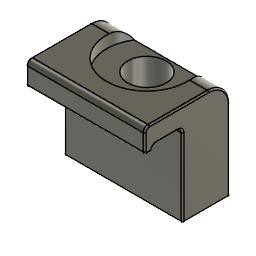
PhoneSupportTop (Autodesk Fusion 360 design; units mm, degrees)
part number: 2026-05-26-19-53-29-844
Autodesk Fusion 360 part; units mm, degrees
sketch "PhoneSupportTop" plane through (0, 0, 0) normal (1, 0, 0) x (0, 1, 0)
  line L0 (0, 0) -> (20, 0)
  line L1 (0, 33) -> (0, 0)
  line L2 (-2, 35) -> (-11, 35)
  line L3 (-13.4495, 33) -> (-15, 33)
  line L4 (-16, 34) -> (-16, 41)
  arc A0 (-11, 35) -> (-12.9596, 33.4) centre (-11, 33) ccw
  arc A1 (0, 33) -> (-2, 35) centre (-2, 33) ccw
  line L5 (-14, 43) -> (11, 43)
  line L6 (20, 0) -> (20, 34)
  arc A2 (20, 34) -> (11, 43) centre (11, 34) ccw
  arc A3 (-14, 43) -> (-16, 41) centre (-14, 41) ccw
  arc A4 (-13.4495, 33) -> (-12.9596, 33.4) centre (-13.4495, 33.5) ccw
  arc A5 (-16, 34) -> (-15, 33) centre (-15, 34) ccw
  point P0 (-13, 33)
  point P1 (-16, 33)
  point P2 (-16, 43)
  dimension "d3" = 20
  dimension "d7" = 4
  dimension "d8" = 3
  dimension "d10" = 2
  dimension "d11" = 9
  dimension "d13" = 34
  dimension "d14" = 27
  dimension "d15" = 10
  dimension "d16" = 9
  dimension "d17" = 2
  dimension "d18" = 0.5
  dimension "d19" = 1
  constraint horizontal L0
  constraint vertical L1
  constraint coincident L0.start L1.end
  constraint perpendicular L1 L2
  constraint horizontal L3
  constraint perpendicular L3 L4
  constraint tangent L1 A1
  constraint tangent L2 A1
  constraint perpendicular L5 L6
  constraint tangent L6 A2
  constraint tangent L5 A2
  constraint coincident P2 L4
  constraint coincident P2 L5
  constraint tangent L4 A3
  constraint tangent L5 A3
  constraint coincident P0 L3
  constraint coincident P0 A0
  constraint tangent L3 A4
  constraint tangent A0 A4
  constraint coincident P1 L3
  constraint coincident P1 L4
  constraint tangent L3 A5
  constraint tangent L4 A5
  measures "d3" distance of L0.start L0.end
  measures "d7" diameter of A0
  measures "d8" distance of P0 P1
  measures "d10" radius of A1
  measures "d11" radius of A2
  measures "d13" distance of L0.end L6.end
  measures "d14" distance of P2 L5.end
  measures "d15" distance of P1 P2
  measures "d16" distance of A0.centre A1.centre
  measures "d17" radius of A3
  measures "d18" radius of A4
  measures "d19" radius of A5
extrude "Extrude1" add sketch "PhoneSupportTop" along normal mid plane 50
sketch "Sketch2" plane through (0, 0, 0) normal (0, 0, 1) x (1, 0, 0)
  line L0 (25, 20) -> (-25, 20) construction
  line L1 (-25, 20) -> (-25, 0) construction
  line L2 (-25, 0) -> (25, 0) construction
  line L3 (25, 0) -> (25, 20) construction
  line L4 (25, 10) -> (-25, 10) construction
  circle A0 centre (0, 10) radius 8.1
  circle A1 centre (16, 10) radius 4.5
  circle A2 centre (-16, 10) radius 4.5
  circle A3 centre (0, 10) radius 17
  dimension "d23" = 16.2
  dimension "d24" = 9
  dimension "d25" = 9
  dimension "d27" = 9
  dimension "d28" = 9
  dimension "d40" = 34
  constraint horizontal L0
  constraint vertical L1
  constraint horizontal L2
  constraint vertical L3
  constraint midpoint L3 L4.start
  constraint midpoint L1 L4.end
  constraint midpoint L4 A0.centre
  constraint coincident L4 A1.centre
  constraint coincident L4 A2.centre
  constraint concentric A0 A3
  measures "d23" diameter of A0
  measures "d24" diameter of A1
  measures "d25" diameter of A2
  measures "d27" horizontal distance of L0.start A1.centre
  measures "d28" horizontal distance of L0.end A2.centre
  measures "d40" diameter of A3
extrude "Extrude2" cut sketch "Sketch2" along normal blind 10 contours A1 A3 | A1 A3 | A2 A3 | A2 A3
extrude "Extrude3" cut sketch "Sketch2" along normal through all contours A0
extrude "Extrude4" cut sketch "Sketch2" against normal blind 5 from surface at 43 contours A1 A2 A3
fillet "Fillet1" radius 0.6 28 edges at (25, 20, 17) (25, 17.364, 40.364) (25, -1.5, 43) (25, -15.4142, 42.4142) (25, -16, 37.5) (25, -15.7071, 33.2929) (25, -14.2247, 33) (25, -13.1333, 33.1127) (25, -12.2649, 34.5492) (25, -6.5, 35) (25, -0.5858, 34.4142) (25, 0, 16.5) (25, 10, 0) (0, 0, 0) (-25, 0, 16.5) (-25, -0.5858, 34.4142) (-25, -6.5, 35) (-25, -12.2649, 34.5492) (-25, -13.1333, 33.1127) (-25, -14.2247, 33) (-25, -15.7071, 33.2929) (-25, -16, 37.5) (-25, -15.4142, 42.4142) (-25, -1.5, 43) (-25, 17.364, 40.364) (-25, 20, 17) (-25, 10, 0) (0, 20, 0)
extrude "Extrude5" cut sketch "Sketch2" against normal blind 5 from surface at 43 contours A1 A3 | A1 A2 A3 | A2 A3 picked at (15.2408, 11.0328) picked at (-15.34, 11.5418)
equation "PhoneSupportThickness = 50 mm"
equation "d21 = PhoneSupportThickness / 2"
equation "d23 = 16 mm + 2 * Tolerance"
equation "Tolerance = 0.1 mm"
named bodies: "PhoneSupportTop"
